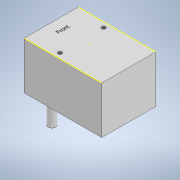
# Autodesk Inventor part: Pump
Saved by Autodesk Inventor 2020 (Build 240168000, 168)
## iProperties
Created: 2020-01-26
Part Number: Pump
Material: Generic
Document SubType Name: Modeling
Designer: holtat
Density: 1 g/cm^3
Appearance: Default
Author: holtat
Autodesk Inventor part; units mm, degrees
ref_plane "YZ Plane" through (0, 0, 0) normal (1, 0, 0) x (0, 1, 0)
ref_plane "XZ Plane" through (0, 0, 0) normal (0, 1, 0) x (-1, 0, 0)
ref_plane "XY Plane" through (0, 0, 0) normal (0, 0, 1) x (1, 0, 0)
sketch "Sketch1" plane through (0, 0, 0) normal (0, 1, 0) x (-1, 0, 0)
  line L0 (32.258, -22.4282) -> (-32.258, -22.4282)
  line L1 (-32.258, -22.4282) -> (-32.258, 22.4282)
  line L2 (-32.258, 22.4282) -> (32.258, 22.4282)
  line L3 (32.258, 22.4282) -> (32.258, -22.4282)
  circle A0 centre (6.858, -18.161) radius 1.5875
  circle A1 centre (6.858, 18.161) radius 1.5875
  line L4 (6.858, -18.161) -> (6.858, 18.161) construction
  point P0 (0, 0)
  point P1 (32.258, 0)
  point P2 (0, -22.4282)
  point P3 (6.858, 0)
  dimension "d0" = 64.516
  dimension "d1" = 44.8564
  dimension "d2" = 3.175
  dimension "d3" = 25.4
  dimension "d4" = 39.116
  dimension "d15" = 36.322
  constraints: 10 end point, 3 midpoint, 2 centre point, 2 horizontal alignment, 2 parallel, 2 vertical alignment, 1 equal radius, 1 horizontal, 1 perpendicular, 1 vertical
  measures "d0" distance between parallel lines of L1 L3
  measures "d1" distance of L2.end L0.start
  measures "d2" diameter of A0
  measures "d3" distance from line of L3 L4.start
  measures "d4" distance from line of L1 L4.start
  measures "d15" distance of L4.end L4.start
extrude "Extrusion1" add sketch "Sketch1" along normal blind 39.37
sketch "Sketch2" plane through (0, 39.37, 0) normal (0, 1, 0) x (1, 0, 0)
  line L0 (-24.1562, -22.4282) -> (-24.1562, 22.4282) construction
  line L1 (-24.1562, 22.4282) -> (-18.3585, 22.4282) construction
  line L2 (-18.3585, 22.4282) -> (-18.3585, -22.4282) construction
  line L3 (-18.3585, -22.4282) -> (-24.1562, -22.4282) construction
  line L4 (32.258, 22.4282) -> (-32.258, 22.4282) projected
  line L5 (-32.258, -22.4282) -> (32.258, -22.4282) projected
  point P0 (0, 0)
  constraints: 2 point on line, 1 vertical alignment, 2 other
sketch "Sketch4" plane through (0, 0, 0) normal (0, -1, 0) x (1, 0, 0)
  circle A0 centre (-23.0124, -8.636) radius 3.175
  circle A1 centre (-23.0124, 8.636) radius 3.175
  line L0 (-32.258, -22.4282) -> (-32.258, 22.4282) projected
  circle A2 centre (-6.858, -18.161) radius 1.5875 projected
  line L1 (-23.0124, -8.636) -> (-23.0124, 8.636) construction
  point P0 (0, 0)
  point P1 (-23.0124, 0)
  dimension "d11" = 17.272
  dimension "d12" = 9.2456
  dimension "d13" = 6.35
  dimension "d14" = 25.4
  constraints: 2 centre point, 2 end point, 1 equal radius, 1 horizontal alignment, 1 midpoint, 1 vertical, 1 vertical alignment
  measures "d11" distance of L1.start L1.end
  measures "d12" distance between parallel lines of L0 L1
  measures "d13" diameter of A0
  measures "d14" distance from line of A2.centre L0
extrude "Extrusion2" add sketch "Sketch4" along normal blind 25.4 contours A0 | A1
body "Solid1"
